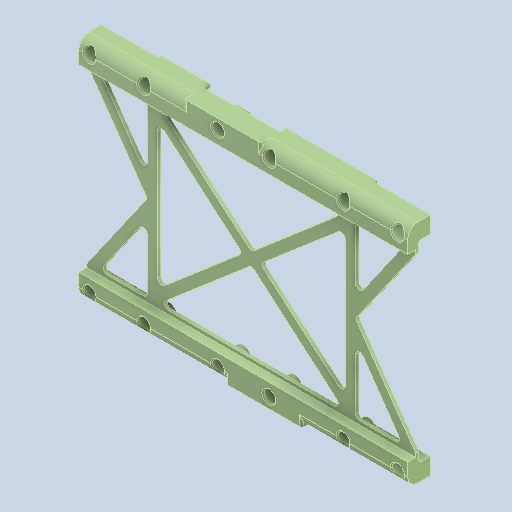
# Autodesk Inventor part: BodyStructure Centre Bottom
Saved by Autodesk Inventor 2023 (Build 270158000, 158)
## iProperties
Created: 2019-11-07
Part Number: BodyStructure Centre Bottom
Material: solidworks materials|ABS
Document SubType Name: Modeling
Designer: Jochen
Density: 1.02 g/cm^3
Appearance: 151,157,178
Sending System: SolidWorks 2017
Last Author: Felix
Last Saved: 2021-02-23
Author: Jochen
Autodesk Inventor part; units mm, degrees
ref_plane "YZ Plane" through (0, 0, 0) normal (1, 0, 0) x (0, 1, 0)
ref_plane "XZ Plane" through (0, 0, 0) normal (0, 1, 0) x (-1, 0, 0)
ref_plane "Work Plane1" through (0, 0, 30) normal (0, 0, 1) x (1, 0, 0)
sketch "Sketch1" plane through (0, 0, 30) normal (0, 0, 1) x (1, 0, 0)
  line L0 (-80, -55) -> (80, -55)
  line L1 (80, 55) -> (-80, 55)
  line L2 (80, 42) -> (80, 42)
  line L3 (0, -77.5799) -> (0, 77.5799) construction
  line L4 (-112, 0) -> (112, 0) construction
  line L5 (-50.649, -42) -> (-50.649, -8.7287)
  line L6 (-45.649, 35.4185) -> (-45.649, -35.4185)
  line L7 (-50.649, -8.7287) -> (-73.9001, -42)
  line L8 (-80, -42) -> (-50.649, 0)
  line L9 (50.649, -8.7287) -> (73.9001, -42)
  line L10 (50.649, -42) -> (50.649, -8.7287)
  line L11 (45.649, 35.4185) -> (45.649, -35.4185)
  line L12 (80, -42) -> (50.649, 0)
  line L13 (50.649, 8.7287) -> (73.9001, 42)
  line L14 (80, 42) -> (50.649, 0)
  line L15 (50.649, 0) -> (50.649, 0)
  line L16 (50.649, 8.7287) -> (50.649, 42)
  line L17 (-50.649, 0) -> (-50.649, 0)
  line L18 (-80, 42) -> (-50.649, 0)
  line L19 (-50.649, 8.7287) -> (-73.9001, 42)
  line L20 (-80, 42) -> (-80, 42)
  line L21 (-50.649, 8.7287) -> (-50.649, 42)
  line L22 (73.9001, 42) -> (50.649, 42)
  line L23 (-73.9001, 42) -> (-50.649, 42)
  line L24 (-45.649, 42) -> (45.649, 42)
  line L25 (-80, -42) -> (-80, -42)
  line L26 (-50.649, -42) -> (-73.9001, -42)
  line L27 (45.649, -42) -> (-45.649, -42)
  line L28 (80, -42) -> (80, -42)
  line L29 (73.9001, -42) -> (50.649, -42)
  line L30 (80, -55) -> (80, -42)
  line L31 (80, 42) -> (80, 55)
  line L32 (-80, 55) -> (-80, 42)
  line L33 (-80, -42) -> (-80, -55)
  line L34 (-48.149, 55) -> (-48.149, -55) construction
  line L35 (-45.649, 42) -> (0, 2.9266)
  line L36 (0, 2.9266) -> (45.649, 42)
  line L37 (45.649, 35.4185) -> (4.2699, 0)
  line L38 (45.649, -35.4185) -> (4.2699, 0)
  line L39 (0, -2.9266) -> (45.649, -42)
  line L40 (-4.2699, 0) -> (-45.649, 35.4185)
  line L41 (-4.2699, 0) -> (-45.649, -35.4185)
  line L42 (0, -2.9266) -> (-45.649, -42)
  point P0 (0, 0)
  point P1 (-2.5, 42)
  point P2 (2.5, 42)
  point P3 (2.5, -42)
  point P4 (-2.5, -42)
  point P5 (50.649, 0)
  point P6 (-50.649, 0)
  dimension "d2" = 5
  dimension "d3" = 0
  dimension "d4" = 160
  dimension "d5" = 13
  dimension "d7" = 110
  dimension "d101" = 5
  dimension "d107" = 5
  constraints: 82 end point, 17 parallel, 15 collinear, 15 perpendicular, 11 point on line, 9 horizontal, 2 vertical, 19 other
  measures "d2" distance between parallel lines of L6 L5
  measures "d3" distance of L8.start L25.end
  measures "d4" distance of L0.start L0.end
  measures "d5" distance of L25.end L0.start
  measures "d7" distance between parallel lines of L1 L0
  measures "d101" distance between parallel lines of L8 L7
  measures "d107" distance between parallel lines of L42 L41
extrude "Extrusion1" add sketch "Sketch1" along normal blind 15.5
fillet "Fillet1" radius 2 22 edges at (-50.649, -42, 37.75) (-50.649, -8.7287, 37.75) (-73.9001, -42, 37.75) (-73.9001, 42, 37.75) (-50.649, 42, 37.75) (-50.649, 8.7287, 37.75) (50.649, -8.7287, 37.75) (50.649, -42, 37.75) (50.649, 42, 37.75) (50.649, 8.7287, 37.75) (73.9001, 42, 37.75) (73.9001, -42, 37.75) (-45.649, 35.4185, 37.75) (0, -2.9266, 37.75) (4.2699, 0, 37.75) (0, 2.9266, 37.75) (-4.2699, 0, 37.75) (-45.649, -35.4185, 37.75) (45.649, -35.4185, 37.75) (45.649, 35.4185, 37.75) (50.649, 0, 37.75) (-50.649, 0, 37.75)
fillet "Fillet1" radius 2 4 edges at (-45.649, 42, 37.75) (-45.649, -42, 37.75) (45.649, -42, 37.75) (45.649, 42, 37.75)
sketch "Sketch3" plane through (0, 0, 0) normal (1, 0, 0) x (0, 1, 0)
  line L0 (0, -10.1) -> (0, 60.6) construction
  line L1 (-77.5799, 0) -> (77.5799, 0) construction
  line L2 (-42, 45.5) -> (-55, 45.5) construction
  line L3 (-55, 45.5) -> (-42, 45.5) construction
  line L4 (-42, 45.5) -> (-1.1456, 45.5) construction
  line L5 (1.1456, 45.5) -> (42, 45.5) construction
  line L6 (42, 45.5) -> (55, 45.5) construction
  line L7 (55, 45.5) -> (42, 45.5) construction
  line L8 (42, 45.5) -> (1.1456, 45.5) construction
  line L9 (-1.1456, 45.5) -> (-42, 45.5) construction
  line L10 (13.9365, 45.5) -> (38.8544, 45.5) construction
  line L11 (42, 45.5) -> (38.8544, 45.5) construction
  line L12 (40, 45.5) -> (42, 45.5) construction
  line L13 (40, 45.5) -> (15.0821, 45.5) construction
  line L14 (13.9365, 45.5) -> (15.0821, 45.5) construction
  line L15 (15.0821, 45.5) -> (40, 45.5) construction
  line L16 (42, 45.5) -> (40, 45.5) construction
  line L17 (38.8544, 45.5) -> (42, 45.5) construction
  line L18 (38.8544, 45.5) -> (13.9365, 45.5) construction
  line L19 (15.0821, 45.5) -> (13.9365, 45.5) construction
  line L20 (-13.9365, 45.5) -> (-38.8544, 45.5) construction
  line L21 (-40, 45.5) -> (-42, 45.5) construction
  line L22 (-40, 45.5) -> (-15.0821, 45.5) construction
  line L23 (-13.9365, 45.5) -> (-15.0821, 45.5) construction
  line L24 (-38.8544, 45.5) -> (-42, 45.5) construction
  line L25 (-38.8544, 45.5) -> (-13.9365, 45.5) construction
  line L26 (-15.0821, 45.5) -> (-13.9365, 45.5) construction
  line L27 (-15.0821, 45.5) -> (-40, 45.5) construction
  line L28 (-42, 45.5) -> (-40, 45.5) construction
  line L29 (-42, 30) -> (-55, 30) construction
  line L30 (-1.1456, 30) -> (-42, 30) construction
  line L31 (42, 30) -> (1.1456, 30) construction
  line L32 (55, 30) -> (42, 30) construction
  line L33 (42, 30) -> (55, 30) construction
  line L34 (1.1456, 30) -> (42, 30) construction
  line L35 (-42, 30) -> (-1.1456, 30) construction
  line L36 (-55, 30) -> (-42, 30) construction
  line L37 (15.0821, 30) -> (13.9365, 30) construction
  line L38 (40, 30) -> (15.0821, 30) construction
  line L39 (42, 30) -> (40, 30) construction
  line L40 (38.8544, 30) -> (42, 30) construction
  line L41 (13.9365, 30) -> (38.8544, 30) construction
  line L42 (13.9365, 30) -> (15.0821, 30) construction
  line L43 (38.8544, 30) -> (13.9365, 30) construction
  line L44 (42, 30) -> (38.8544, 30) construction
  line L45 (40, 30) -> (42, 30) construction
  line L46 (15.0821, 30) -> (40, 30) construction
  line L47 (-15.0821, 30) -> (-13.9365, 30) construction
  line L48 (-40, 30) -> (-15.0821, 30) construction
  line L49 (-42, 30) -> (-40, 30) construction
  line L50 (-13.9365, 30) -> (-38.8544, 30) construction
  line L51 (-40, 30) -> (-42, 30) construction
  line L52 (-15.0821, 30) -> (-40, 30) construction
  line L53 (-13.9365, 30) -> (-15.0821, 30) construction
  line L54 (-38.8544, 30) -> (-13.9365, 30) construction
  line L55 (-42, 30) -> (-38.8544, 30) construction
  line L56 (55, 30) -> (55, 45.5) construction
  line L57 (55, 30) -> (55, 45.5) construction
  line L58 (-55, 30) -> (-55, 45.5) construction
  line L59 (-55, 30) -> (-55, 45.5) construction
  line L60 (-37, 30) -> (-37, 45.5) construction
  line L61 (-37, 30) -> (-37, 45.5) construction
  line L62 (-55, 30) -> (-55, 40.5)
  line L63 (-47.5, 45.5) -> (-45, 45.5)
  line L64 (-43.75, 41.5) -> (43.75, 41.5)
  line L65 (55, 40.5) -> (55, 30)
  line L66 (55, 30) -> (-55, 30)
  line L67 (-46.25, 45.5) -> (-46.25, 30) construction
  line L68 (-38.8544, 30) -> (-42, 30) projected
  line L69 (-42, 45.5) -> (-38.8544, 45.5) projected
  line L70 (42, 45.5) -> (42, 30) projected
  line L71 (42, 30) -> (42, 45.5) projected
  line L72 (1.1456, 30) -> (-1.1456, 30) projected
  line L73 (-1.1456, 30) -> (1.1456, 30) projected
  line L74 (1.1456, 45.5) -> (-1.1456, 45.5) projected
  line L75 (-1.1456, 45.5) -> (1.1456, 45.5) projected
  line L76 (-55, 45.5) -> (-55, 40.5) construction
  line L77 (-43.75, 41.5) -> (-43.75, 45.5)
  line L78 (-43.75, 45.5) -> (-45, 45.5)
  line L79 (-55, 45.5) -> (-42, 45.5) projected
  line L80 (-47.5, 45.5) -> (-55, 45.5)
  line L81 (-55, 30) -> (-55, 45.5) projected
  arc A0 (-50, 45.5) -> (-55, 40.5) centre (-50, 40.5) ccw
  line L82 (42, 45.5) -> (55, 45.5) projected
  arc A1 (55, 40.5) -> (50, 45.5) centre (50, 40.5) ccw
  line L83 (43.75, 41.5) -> (43.75, 45.5)
  line L84 (50, 45.5) -> (43.75, 45.5)
  point P0 (0, 0)
  point P1 (-55, 35.25)
  point P2 (-50, 45.5)
  dimension "d113" = 5
  dimension "d114" = 4
  dimension "d115" = 87.5
  constraints: 27 end point, 6 point on line, 4 perpendicular, 4 point on circle, 4 tangent, 3 collinear, 2 centre point, 2 horizontal, 2 midpoint, 2 vertical, 1 equal radius, 1 parallel, 7 other
  measures "d113" radius of A0
  measures "d114" distance of L64.start L77.end
  measures "d115" distance between parallel lines of L77 L83
extrude "Extrusion3" cut sketch "Sketch3" along normal through all both and the other way through all contours L62 A0 L79 L63 L78 L77 L64 L70 L66 | L70 L64 L83 L82 A1 L65 L66 keep common part
sketch "Sketch12" plane through (80, -55, 30) normal (1, 0, 0) x (0, 0, -1)
  line L0 (0, 13) -> (0, 0) projected
  line L1 (0, 0) -> (-10.5, 0) projected
  line L2 (-10.5, 110) -> (0, 110) projected
  line L3 (0, 110) -> (0, 97) projected
  line L4 (-11.5, 13) -> (0, 13) projected
  line L5 (0, 97) -> (-11.5, 97) projected
  line L6 (-11.5, 97) -> (-11.5, 98.75) projected
  line L7 (-11.5, 98.75) -> (-15.5, 98.75) projected
  line L8 (-15.5, 98.75) -> (-15.5, 105) projected
  arc A0 (-10.5, 110) -> (-15.5, 105) centre (-10.5, 105) ccw projected
  arc A1 (-15.5, 5) -> (-10.5, 0) centre (-10.5, 5) ccw projected
  line L9 (-15.5, 5) -> (-15.5, 11.25) projected
  line L10 (-15.5, 11.25) -> (-11.5, 11.25) projected
  line L11 (-11.5, 11.25) -> (-11.5, 13) projected
  point P0 (30, 55)
  point P1 (-11.5, 11.4559)
  point P2 (-11.5, 98.5441)
sketch "Sketch15" plane through (0, 0, 0) normal (0, 1, 0) x (-1, 0, 0)
  line L0 (-51.089, 41.5) -> (-45.649, 41.5) construction
  line L1 (-45.649, 41.5) -> (-45.649, 30) construction
  line L2 (-45.649, 30) -> (-51.089, 30) construction
  line L3 (-51.089, 30) -> (-51.089, 41.5) construction
  line L4 (-5.3456, 41.5) -> (5.3456, 41.5) construction
  line L5 (5.3456, 41.5) -> (5.3456, 30) construction
  line L6 (5.3456, 30) -> (-5.3456, 30) construction
  line L7 (-5.3456, 30) -> (-5.3456, 41.5) construction
  line L8 (45.649, 41.5) -> (51.089, 41.5) construction
  line L9 (51.089, 41.5) -> (51.089, 30) construction
  line L10 (51.089, 30) -> (45.649, 30) construction
  line L11 (45.649, 30) -> (45.649, 41.5) construction
  line L12 (-27.5, 45.5) -> (-8.5, 45.5)
  line L13 (-8.5, 44.5) -> (-8.5, 30)
  line L14 (-8.5, 30) -> (-28.5, 30)
  line L15 (-28.5, 30) -> (-28.5, 44.5)
  line L16 (-8.5, 30) -> (8.5, 30)
  line L17 (8.5, 30) -> (8.5, 44.5)
  line L18 (7.5, 45.5) -> (-7.5, 45.5)
  line L19 (-8.5, 45.5) -> (-8.5, 30)
  line L20 (8.5, 30) -> (28.5, 30)
  line L21 (28.5, 30) -> (28.5, 44.5)
  line L22 (27.5, 45.5) -> (8.5, 45.5)
  line L23 (8.5, 45.5) -> (8.5, 30)
  line L24 (80, 45.5) -> (-80, 45.5) construction
  line L25 (-42.3485, 30) -> (-6.0451, 30) construction
  arc A0 (-27.5, 45.5) -> (-28.5, 44.5) centre (-27.5, 44.5) ccw
  arc A1 (28.5, 44.5) -> (27.5, 45.5) centre (27.5, 44.5) ccw
  arc A2 (8.5, 44.5) -> (7.5, 45.5) centre (7.5, 44.5) ccw
  arc A3 (-7.5, 45.5) -> (-8.5, 44.5) centre (-7.5, 44.5) ccw
  line L26 (-8.5, 45.5) -> (-7.5, 45.5)
  line L27 (7.5, 45.5) -> (8.5, 45.5)
  line L28 (28.5, 36.2) -> (-28.5, 36.2)
  point P0 (0, 0)
  point P1 (-28.5, 45.5)
  point P2 (28.5, 45.5)
  point P3 (28.5, 37.25)
  point P4 (-8.5, 36.2)
  point P5 (8.5, 36.2)
  dimension "d123" = 37
  dimension "d124" = 37
  dimension "d125" = 51.5
  dimension "d126" = 51.5
  dimension "d131" = 1
  dimension "d133" = 9.3
  constraints: 30 end point, 16 point on line, 10 tangent, 9 point on circle, 6 parallel, 4 centre point, 4 horizontal, 3 equal radius, 3 perpendicular, 2 collinear, 1 midpoint
  measures "d123" distance between parallel lines of L17 L15
  measures "d124" distance from line of point (28.5, 37.25) L13
  measures "d125" distance from line of L15 L24.end
  measures "d126" horizontal distance of L24.start L20.end
  measures "d131" radius of A0
  measures "d133" distance between parallel lines of L28 L24
extrude "Extrusion12" add sketch "Sketch15" against normal blind 10 from surface at 55 contours A3 L18 A2 L17 L28 L13 | L28 L17 L16 L13 | L27 L23 A2 | L28 L21 L20 L17 | L17 L23 L22 A1 L21 L28
extrude "Extrusion13" add sketch "Sketch15" along normal blind 10 from surface at -55 contours L12 L19 L13 L28 L15 A0 | L26 A3 L19 | A3 L18 A2 L17 L28 L13 | L28 L13 L14 L15 | L28 L17 L16 L13
sketch "Sketch5" plane through (0, 0, 0) normal (0, 1, 0) x (-1, 0, 0)
  line L0 (114, 0) -> (-124, 0) construction
  line L1 (0, -9.1) -> (0, 54.6) construction
  line L2 (80, 41.5) -> (80, 45.5) construction
  line L3 (-80, 30) -> (-80, 40.5) construction
  line L4 (-80, 30) -> (80, 30) construction
  line L5 (80, 30) -> (80, 40.5) construction
  line L6 (80, 39.5) -> (80, 41.5) construction
  line L7 (-80, 41.5) -> (-80, 39.5) construction
  line L8 (-52, 40) -> (-52, 33)
  line L9 (-52, 33) -> (-45, 33)
  line L10 (-45, 33) -> (-45, 40)
  line L11 (-45, 40) -> (-16, 40)
  line L12 (-16, 40) -> (-16, 33)
  line L13 (-16, 33) -> (-9, 33)
  line L14 (-9, 33) -> (-9, 40)
  line L15 (-9, 40) -> (9, 40)
  line L16 (9, 40) -> (9, 33)
  line L17 (9, 33) -> (16, 33)
  line L18 (16, 33) -> (16, 40)
  line L19 (16, 40) -> (45, 40)
  line L20 (45, 40) -> (45, 33)
  line L21 (45, 33) -> (52, 33)
  line L22 (52, 33) -> (52, 40)
  line L23 (80, 34.5) -> (80, 45.5)
  line L24 (80, 30) -> (-80, 30) construction
  line L25 (-80, 45.5) -> (-80, 34.5)
  line L26 (80, 41.5) -> (-80, 41.5)
  line L27 (52, 34.5) -> (80, 34.5)
  line L28 (-80, 34.5) -> (-52, 34.5)
  line L29 (52, 40) -> (45, 40) construction
  line L30 (-8.5, 40.5) -> (-80, 40.5) projected
  line L31 (80, 45.5) -> (-80, 45.5) projected
  line L32 (-80, 45.5) -> (80, 45.5)
  line L33 (80, 40.5) -> (28.5, 40.5) projected
  line L34 (-7.5, 45.5) -> (27.5, 45.5) projected
  line L35 (28.5, 44.5) -> (28.5, 40.5) projected
  arc A0 (28.5, 44.5) -> (27.5, 45.5) centre (27.5, 44.5) ccw projected
  arc A1 (-7.5, 45.5) -> (-8.5, 44.5) centre (-7.5, 44.5) ccw projected
  line L36 (-8.5, 40.5) -> (-8.5, 44.5) projected
  point P0 (0, 0)
  point P1 (61.4737, 40)
  point P2 (56.7369, 40)
  point P3 (48.5, 33)
  dimension "d47" = 7
  dimension "d48" = 9
  dimension "d51" = 11
  dimension "d96" = 7
  dimension "d102" = 48.5
  dimension "d118" = 12.5
  constraints: 44 end point, 14 point on line, 10 perpendicular, 4 collinear, 1 horizontal, 1 midpoint, 1 parallel, 1 vertical, 2 other
  measures "d47" distance between parallel lines of L22 L20
  measures "d48" distance between parallel lines of L1 L16
  measures "d51" distance from line of L2.end L27
  measures "d96" distance between parallel lines of L21 L29
  measures "d102" distance from line of L1 point (48.5, 33)
  measures "d118" distance between parallel lines of L31 L13
extrude "Extrusion5" cut sketch "Sketch5" along normal through all both and the other way through all keep common part
sketch "Sketch6" plane through (0, 0, 0) normal (1, 0, 0) x (0, 1, 0)
  line L0 (0, -9.1) -> (0, 54.6) construction
  line L1 (-77.5799, 0) -> (77.5799, 0) construction
  line L2 (-38.535, 41.5) -> (-36.9915, 41.5) construction
  line L3 (-46.875, 40) -> (-46.875, 25)
  line L4 (-46.875, 25) -> (46.875, 25)
  line L5 (46.875, 25) -> (46.875, 40)
  line L6 (-46.875, 40) -> (46.875, 40)
  line L7 (42, 40) -> (55, 40) projected
  line L8 (-43.75, 45.5) -> (-50, 45.5) construction
  line L9 (46.875, 25) -> (54.125, 25)
  line L10 (54.125, 25) -> (54.125, 40)
  line L11 (46.875, 40) -> (54.125, 40)
  line L12 (-46.875, 40) -> (-54.125, 40)
  line L13 (-54.125, 40) -> (-54.125, 25)
  line L14 (-54.125, 25) -> (-46.875, 25)
  line L15 (55, 33) -> (55, 40) projected
  line L16 (55, 33) -> (55, 25)
  line L17 (55, 25) -> (54.125, 25)
  line L18 (55, 33) -> (55, 40)
  line L19 (55, 40) -> (54.125, 40)
  line L20 (-54.125, 25) -> (-55, 25)
  line L21 (-55, 25) -> (-55, 40)
  line L22 (-55, 40) -> (-54.125, 40)
  point P0 (0, 0)
  point P1 (-46.875, 32.5)
  point P2 (54.9365, 40)
  point P3 (-45, 45.5)
  point P4 (-47.5, 45.5)
  point P5 (-46.875, 45.5)
  point P6 (55, 39.5)
  point P7 (-55, 33)
  point P8 (55, 39.5)
  point P9 (54.9365, 40)
  point P10 (-54.9365, 40)
  point P11 (-54.9161, 45.5)
  point P12 (54.9791, 40)
  point P13 (-42, 45.5)
  point P14 (-55, 45.5)
  dimension "d75" = 1.5
  dimension "d104" = 15
  dimension "d106" = 7.25
  constraints: 37 end point, 6 perpendicular, 6 point on line, 4 collinear, 2 horizontal, 2 midpoint, 2 vertical, 1 parallel, 1 other
  measures "d75" distance between parallel lines of L6 L2
  measures "d104" distance from line of L6 L3.end
  measures "d106" distance between parallel lines of L5 L10
extrude "Extrusion6" cut sketch "Sketch6" along normal mid plane 160 contours L6 L5 L4 L3
sketch "Sketch9" plane through (45, -54.9365, 40) normal (0, 0, -1) x (-1, 0, 0)
  line L0 (-35, 101.8115) -> (-35, 109.9365) projected
  line L1 (-35, -0.0635) -> (-35, 8.0615) projected
  line L2 (125, 109.9365) -> (125, 101.8115) projected
  line L3 (125, 8.0615) -> (125, -0.0635) projected
  circle A0 centre (-30, 104.9365) radius 1.5
  circle A1 centre (32.5, 104.9365) radius 1.5
  circle A2 centre (-3.5, 104.9365) radius 1.5
  circle A3 centre (57.5, 104.9365) radius 1.5
  circle A4 centre (93.5, 104.9365) radius 1.5
  circle A5 centre (120, 104.9365) radius 1.5
  circle A6 centre (120, 4.9365) radius 1.5
  circle A7 centre (93.5, 4.9365) radius 1.5
  circle A8 centre (57.5, 4.9365) radius 1.5
  circle A9 centre (-3.5, 4.9365) radius 1.5
  circle A10 centre (32.5, 4.9365) radius 1.5
  circle A11 centre (-30, 4.9365) radius 1.5
  line L4 (-30, 104.9365) -> (120, 104.9365) construction
  line L5 (120, 104.9365) -> (120, 4.9365) construction
  line L6 (120, 4.9365) -> (-30, 4.9365) construction
  line L7 (-30, 4.9365) -> (-30, 104.9365) construction
  line L8 (157, 54.9365) -> (-67, 54.9365) construction
  line L9 (45, -23.5133) -> (45, 133.3862) construction
  line L10 (32.5, 104.9365) -> (32.5, 4.9365) construction
  line L11 (-3.5, 4.9365) -> (-3.5, 104.9365) construction
  line L12 (93.5, 104.9365) -> (93.5, 4.9365) construction
  line L13 (57.5, 104.9365) -> (57.5, 4.9365) construction
  circle A12 centre (-30, 4.9365) radius 2.9
  circle A13 centre (-3.5, 4.9365) radius 2.9
  circle A14 centre (32.5, 4.9365) radius 2.9
  circle A15 centre (57.5, 4.9365) radius 2.9
  circle A16 centre (93.5, 4.9365) radius 2.9
  circle A17 centre (120, 4.9365) radius 2.9
  circle A18 centre (120, 104.9365) radius 2.9
  circle A19 centre (93.5, 104.9365) radius 2.9
  circle A20 centre (57.5, 104.9365) radius 2.9
  circle A21 centre (32.5, 104.9365) radius 2.9
  circle A22 centre (-3.5, 104.9365) radius 2.9
  circle A23 centre (-30, 104.9365) radius 2.9
  line L14 (125, 108.4365) -> (-35, 108.4365)
  line L15 (-35, 1.4365) -> (125, 1.4365)
  line L16 (-35, 109.9365) -> (0, 109.9365) projected
  line L17 (0, -0.0635) -> (-35, -0.0635) projected
  line L18 (125, -0.0635) -> (90, -0.0635) projected
  line L19 (90, 109.9365) -> (125, 109.9365) projected
  line L20 (61, 109.9365) -> (61, 101.8115) projected
  line L21 (29, 109.9365) -> (36, 109.9365) projected
  line L22 (54, 109.9365) -> (61, 109.9365) projected
  line L23 (61, -0.0635) -> (54, -0.0635) projected
  line L24 (36, -0.0635) -> (29, -0.0635) projected
  line L25 (90, 8.0615) -> (125, 8.0615) projected
  line L26 (90, -0.0635) -> (90, 8.0615) projected
  line L27 (54, -0.0635) -> (54, 8.0615) projected
  line L28 (36, 8.0615) -> (36, -0.0635) projected
  line L29 (29, -0.0635) -> (29, 8.0615) projected
  line L30 (0, 8.0615) -> (0, -0.0635) projected
  line L31 (125, 101.8115) -> (90, 101.8115) projected
  line L32 (90, 101.8115) -> (90, 109.9365) projected
  line L33 (61, 109.9365) -> (90, 109.9365) projected
  line L34 (36, 109.9365) -> (54, 109.9365) projected
  line L35 (0, 109.9365) -> (29, 109.9365) projected
  line L36 (0, 101.8115) -> (-35, 101.8115) projected
  line L37 (0, 109.9365) -> (0, 101.8115) projected
  line L38 (125, 101.8115) -> (125, 96.9365) projected
  line L39 (61, 101.8115) -> (54, 101.8115) projected
  line L40 (54, 101.8115) -> (54, 109.9365) projected
  line L41 (36, 109.9365) -> (36, 101.8115) projected
  line L42 (36, 101.8115) -> (29, 101.8115) projected
  line L43 (29, 101.8115) -> (29, 109.9365) projected
  line L44 (-35, 96.9365) -> (-35, 101.8115) projected
  line L45 (-6.4496, 56.0821) -> (-35, 96.9365) projected
  arc A24 (-6.4496, 53.7909) -> (-6.4496, 56.0821) centre (-8.089, 54.9365) ccw projected
  line L46 (-35, 12.9365) -> (-6.4496, 53.7909) projected
  line L47 (-35, 8.0615) -> (-35, 12.9365) projected
  line L48 (-35, 8.0615) -> (0, 8.0615) projected
  line L49 (125, 96.9365) -> (96.4496, 56.0821) projected
  arc A25 (96.4496, 56.0821) -> (96.4496, 53.7909) centre (98.089, 54.9365) ccw projected
  line L50 (96.4496, 53.7909) -> (125, 12.9365) projected
  line L51 (125, 12.9365) -> (125, 8.0615) projected
  line L52 (29, -0.0635) -> (0, -0.0635) projected
  line L53 (29, 8.0615) -> (36, 8.0615) projected
  line L54 (54, -0.0635) -> (36, -0.0635) projected
  line L55 (54, 8.0615) -> (61, 8.0615) projected
  line L56 (61, 8.0615) -> (61, -0.0635) projected
  line L57 (90, -0.0635) -> (61, -0.0635) projected
  line L58 (-5.649, 14.9365) -> (-5.649, 39.8543) projected
  arc A26 (-5.649, 39.8543) -> (-9.2884, 41) centre (-7.649, 39.8543) ccw projected
  line L59 (-9.2884, 41) -> (-26.7018, 16.0821) projected
  arc A27 (-26.7018, 16.0821) -> (-25.0624, 12.9365) centre (-25.0624, 14.9365) ccw projected
  line L60 (-25.0624, 12.9365) -> (-7.649, 12.9365) projected
  arc A28 (-7.649, 12.9365) -> (-5.649, 14.9365) centre (-7.649, 14.9365) ccw projected
  line L61 (-5.649, 70.0186) -> (-5.649, 94.9365) projected
  arc A29 (-5.649, 94.9365) -> (-7.649, 96.9365) centre (-7.649, 94.9365) ccw projected
  line L62 (-7.649, 96.9365) -> (-25.0624, 96.9365) projected
  arc A30 (-25.0624, 96.9365) -> (-26.7018, 93.7909) centre (-25.0624, 94.9365) ccw projected
  line L63 (-26.7018, 93.7909) -> (-9.2884, 68.873) projected
  arc A31 (-9.2884, 68.873) -> (-5.649, 70.0186) centre (-7.649, 70.0186) ccw projected
  arc A32 (97.649, 96.9365) -> (95.649, 94.9365) centre (97.649, 94.9365) ccw projected
  line L64 (95.649, 94.9365) -> (95.649, 70.0186) projected
  arc A33 (95.649, 70.0186) -> (99.2884, 68.873) centre (97.649, 70.0186) ccw projected
  line L65 (99.2884, 68.873) -> (116.7018, 93.7909) projected
  arc A34 (116.7018, 93.7909) -> (115.0624, 96.9365) centre (115.0624, 94.9365) ccw projected
  line L66 (115.0624, 96.9365) -> (97.649, 96.9365) projected
  arc A35 (115.0624, 12.9365) -> (116.7018, 16.0821) centre (115.0624, 14.9365) ccw projected
  line L67 (116.7018, 16.0821) -> (99.2884, 41) projected
  arc A36 (99.2884, 41) -> (95.649, 39.8543) centre (97.649, 39.8543) ccw projected
  line L68 (95.649, 39.8543) -> (95.649, 14.9365) projected
  arc A37 (95.649, 14.9365) -> (97.649, 12.9365) centre (97.649, 14.9365) ccw projected
  line L69 (97.649, 12.9365) -> (115.0624, 12.9365) projected
  arc A38 (87.3485, 22.3431) -> (90.649, 23.8625) centre (88.649, 23.8625) ccw projected
  line L70 (90.649, 23.8625) -> (90.649, 86.0105) projected
  arc A39 (90.649, 86.0105) -> (87.3485, 87.5299) centre (88.649, 86.0105) ccw projected
  line L71 (87.3485, 87.5299) -> (51.0451, 56.4559) projected
  arc A40 (51.0451, 56.4559) -> (51.0451, 53.4171) centre (52.3456, 54.9365) ccw projected
  line L72 (51.0451, 53.4171) -> (87.3485, 22.3431) projected
  line L73 (43.6995, 50.8966) -> (3.4627, 16.4559) projected
  arc A41 (3.4627, 16.4559) -> (4.7632, 12.9365) centre (4.7632, 14.9365) ccw projected
  line L74 (4.7632, 12.9365) -> (85.2368, 12.9365) projected
  arc A42 (85.2368, 12.9365) -> (86.5373, 16.4559) centre (85.2368, 14.9365) ccw projected
  line L75 (86.5373, 16.4559) -> (46.3005, 50.8966) projected
  arc A43 (46.3005, 50.8966) -> (43.6995, 50.8966) centre (45, 49.3772) ccw projected
  line L76 (38.9549, 56.4559) -> (2.6515, 87.5299) projected
  arc A44 (2.6515, 87.5299) -> (-0.649, 86.0105) centre (1.351, 86.0105) ccw projected
  line L77 (-0.649, 86.0105) -> (-0.649, 23.8625) projected
  arc A45 (-0.649, 23.8625) -> (2.6515, 22.3431) centre (1.351, 23.8625) ccw projected
  line L78 (2.6515, 22.3431) -> (38.9549, 53.4171) projected
  arc A46 (38.9549, 53.4171) -> (38.9549, 56.4559) centre (37.6544, 54.9365) ccw projected
  line L79 (85.2368, 96.9365) -> (4.7632, 96.9365) projected
  arc A47 (4.7632, 96.9365) -> (3.4627, 93.4171) centre (4.7632, 94.9365) ccw projected
  line L80 (3.4627, 93.4171) -> (43.6995, 58.9763) projected
  arc A48 (43.6995, 58.9763) -> (46.3005, 58.9763) centre (45, 60.4957) ccw projected
  line L81 (46.3005, 58.9763) -> (86.5373, 93.4171) projected
  arc A49 (86.5373, 93.4171) -> (85.2368, 96.9365) centre (85.2368, 94.9365) ccw projected
  line L82 (97.7, 1.4365) -> (97.7, -0.0635)
  line L83 (97.7, 108.4365) -> (97.7, 109.9365)
  line L84 (16.5, -0.0635) -> (-35, -0.0635) projected
  line L85 (-7.7, -0.0635) -> (-7.7, 1.4365)
  line L86 (-7.7, 108.4365) -> (-7.7, 109.9365)
  line L87 (125, 109.9365) -> (-35, 109.9365) projected
  point P0 (45, 54.9365)
  point P1 (42.5, 12.9365)
  point P2 (-6, 80.6486)
  point P3 (-6, 19.2244)
  point P4 (-6, 14.9365)
  point P5 (47.5, 86.9365)
  point P6 (42.5, 76.9365)
  point P7 (42.5, 22.9365)
  point P8 (47.5, 76.9365)
  point P9 (47.5, 22.9365)
  point P10 (-6, 36.0374)
  point P11 (98.4175, 46.8521)
  point P12 (45, 52.0098)
  point P13 (45, 57.8631)
  point P14 (-5.649, 54.9365)
  point P15 (95.649, 54.9365)
  point P16 (1, 109.9365)
  point P17 (28, 109.9365)
  point P18 (37, 109.9365)
  point P19 (53, 109.9365)
  point P20 (62, 109.9365)
  point P21 (89, 109.9365)
  point P22 (98, 109.9365)
  point P23 (89, -0.0635)
  point P24 (62, -0.0635)
  point P25 (53, -0.0635)
  point P26 (37, -0.0635)
  point P27 (28, -0.0635)
  point P28 (1, -0.0635)
  point P29 (-8, -0.0635)
  point P30 (61, 108.4365)
  point P31 (36, 1.4365)
  point P32 (29, 1.4365)
  point P33 (90, 1.4365)
  point P34 (90, 108.4365)
  point P35 (54, 108.4365)
  point P36 (0, 1.4365)
  point P37 (0, 108.4365)
  point P38 (36.5, -0.0635)
  point P39 (16.5, 109.9365)
  dimension "d61" = 3
  dimension "d63" = 100
  dimension "d64" = 75
  dimension "d65" = 48.5
  dimension "d66" = 12.5
  dimension "d69" = 5.8
  dimension "d117" = 1.5
  dimension "d132" = 7.7
  constraints: 28 end point, 24 centre point, 22 equal radius, 19 point on line, 15 coincident, 7 perpendicular, 3 parallel, 2 collinear, 2 vertical, 1 horizontal, 8 other
  measures "d61" diameter of A0
  measures "d63" distance of L6.end L4.start
  measures "d64" distance from line of A11.centre L9
  measures "d65" distance from line of L11.start L9
  measures "d66" distance from line of L10.end L9
  measures "d69" diameter of A12
  measures "d117" distance between parallel lines of L16 L14
  measures "d132" distance between parallel lines of L26 L82
fillet "Fillet5" radius 3.5 16 edges at (-52, -46.875, 33.75) (-45, -46.875, 36.5) (-16, -46.875, 36.5) (-9, -46.875, 36.5) (9, -46.875, 36.5) (16, -46.875, 36.5) (45, -46.875, 36.5) (52, -46.875, 33.75) (52, 46.875, 33.75) (45, 46.875, 36.5) (16, 46.875, 36.5) (9, 46.875, 36.5) (-9, 46.875, 36.5) (-16, 46.875, 36.5) (-45, 46.875, 36.5) (-52, 46.875, 33.75)
fillet "Fillet4" radius 1 12 edges at (9, -52.6874, 40) (9, 52.6874, 40) (16, -52.6874, 40) (16, 52.6874, 40) (45, -52.6874, 40) (45, 52.6874, 40) (-45, -52.6874, 40) (-45, 52.6874, 40) (-16, -52.6874, 40) (-16, 52.6874, 40) (-9, -52.6874, 40) (-9, 52.6874, 40)
extrude "Extrusion8" cut sketch "Sketch9" along normal through all both and the other way through all contours A0 | A1 | A2 | A3 | A4 | A5 | A6 | A7 | A8 | A9 | A10 | A11
extrude "Extrusion9" cut sketch "Sketch9" against normal through all contours A0 | A1 | A2 | A3 | A4 | A5 | A6 | A7 | A8 | A9 | A10 | A11 | A12 | A13 | A14 | A15 | A16 | A17 | A18 | A19 | A20 | A21 | A22 | A23
sketch "Sketch10" plane through (0, 0, 0) normal (1, 0, 0) x (0, 1, 0)
  line L0 (-77.5799, 0) -> (77.5799, 0) construction
  line L1 (0, -9.1) -> (0, 54.6) construction
  line L2 (-43.5, 40) -> (43.5, 40)
  line L3 (43.5, 40) -> (43.5, 34.5)
  line L4 (43.5, 34.5) -> (-43.5, 34.5)
  line L5 (-43.5, 34.5) -> (-43.5, 40)
  line L6 (29.1214, 34.5) -> (55, 34.5) construction
  point P0 (0, 0)
  dimension "d105" = 87
  constraints: 8 end point, 2 parallel, 1 horizontal, 1 perpendicular, 1 point on line, 1 other
  measures "d105" distance of L3.end L4.end
extrude "Extrusion10" cut sketch "Sketch10" along normal through all both and the other way through all
extrude "Extrusion11" add sketch "Sketch9" along normal up to surface (7 mm away) contours L86 L16 L37 L14 | L37 L35 L43 L14 | L43 L21 L41 L14 | L41 L34 L40 L14 | L40 L22 L20 L14 | L20 L33 L32 L14 | L32 L19 L83 L14 | L15 L30 L17 L85 | L15 L29 L52 L30 | L15 L28 L24 L29 | L15 L27 L54 L28 | L15 L56 L23 L27 | L15 L26 L57 L56 | L15 L82 L18 L26 | A13 | A14 | A15 | A16 | A19 | A20 | A22
fillet "Fillet6" radius 0.5 22 edges at (75, 47.1, 45.5) (75.0007, 52.9, 44.5731) (48.5, 47.1, 45.5) (48.5007, 52.9, 44.5731) (12.5007, 52.9, 44.5731) (12.5, 47.1, 45.5) (-9.6, 50, 45.5) (-48.5, 47.1, 45.5) (-48.4993, 52.9, 44.5731) (-75, 47.1, 45.5) (-74.9993, 52.9, 44.5731) (-75.0007, -52.9, 44.5731) (-75, -47.1, 45.5) (-48.5007, -52.9, 44.5731) (-48.5, -47.1, 45.5) (-12.5007, -52.9, 44.5731) (-12.5, -47.1, 45.5) (15.4, -50, 45.5) (48.4993, -52.9, 44.5731) (48.5, -47.1, 45.5) (74.9993, -52.9, 44.5731) (75, -47.1, 45.5)
extrude "Extrusion14" cut sketch "Sketch15" against normal blind 2.2 from surface at 55 contours L28 L17 L16 L13 | L28 L21 L20 L17
extrude "Extrusion15" cut sketch "Sketch15" along normal blind 2.2 from surface at -55 contours L28 L13 L14 L15 | L28 L17 L16 L13
equation "\"d2\" = d1"
equation "\"d1\" = 5"
body "Solid1"
body "Solid2"
